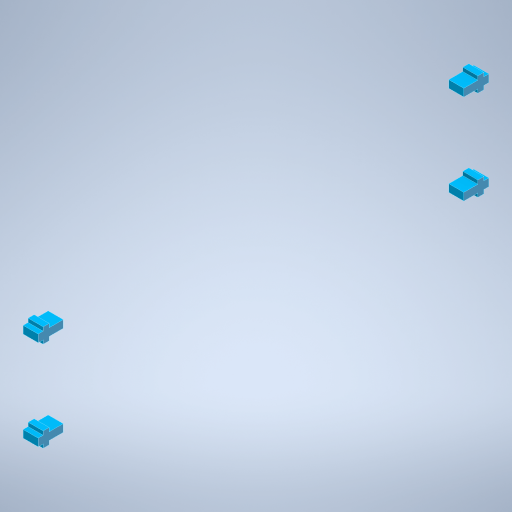
# Autodesk Inventor part: передняя стенка
Saved by Autodesk Inventor 2024.2 (Build 282272000, 272)
## iProperties
Created: 2025-11-20
Part Number: передняя стенка
Material: Типовые
Document SubType Name: Modeling
Designer: Zakhar
Density: 1 g/cm^3
Appearance: Небесно-голубой — нейтральный
Mass: 95.616 g
Surface Area: 351.84 cm^2
Volume: 95.616 cm^3
Author: Zakhar
Autodesk Inventor part; units mm, degrees
ref_plane "YZ Plane" through (0, 0, 0) normal (1, 0, 0) x (0, 1, 0)
ref_plane "XZ Plane" through (0, 0, 0) normal (0, 1, 0) x (-1, 0, 0)
ref_plane "XY Plane" through (0, 0, 0) normal (0, 0, 1) x (1, 0, 0)
sketch "Эскиз1" plane through (0, 0, 0) normal (1, 0, 0) x (0, 1, 0)
  line L0 (84, 90) -> (0, 90)
  line L1 (0, 90) -> (0, -90)
  line L2 (0, -90) -> (84, -90)
  line L3 (84, -90) -> (84, 90)
  line L4 (76, 90) -> (8, 90)
  line L5 (8, 90) -> (8, 96)
  line L6 (8, 96) -> (76, 96)
  line L7 (76, 96) -> (76, 90)
  line L8 (76, -90) -> (8, -90)
  line L9 (8, -90) -> (8, -96)
  line L10 (8, -96) -> (76, -96)
  line L11 (76, -96) -> (76, -90)
  line L12 (16, -96) -> (16, -90)
  line L13 (32, -96) -> (32, -90)
  line L14 (68, -96) -> (68, -90)
  line L15 (52, -96) -> (52, -90)
  line L16 (16, 90) -> (16, 96)
  line L17 (32, 90) -> (32, 96)
  line L18 (68, 90) -> (68, 96)
  line L19 (52, 90) -> (52, 96)
  circle A0 centre (20, -59.5) radius 1.5
  circle A1 centre (20, -73.5) radius 1.5
  circle A2 centre (7, -59.5) radius 1.5
  circle A3 centre (7, -73.5) radius 1.5
  line L20 (20, -59.5) -> (0, -59.5) construction
  line L21 (7, -59.5) -> (7, -73.5) construction
  line L22 (20, -73.5) -> (0, -73.5) construction
  point P0 (0, 0)
  point P1 (76, 93)
  point P2 (8, 93)
  point P3 (8, -90)
  point P4 (68, -93)
  point P5 (76, -93)
  point P6 (52, -93)
  point P7 (16, -93)
  point P8 (8, -93)
  point P9 (32, -93)
  point P10 (68, 93)
  point P11 (52, 93)
  point P12 (16, 93)
  point P13 (32, 93)
  dimension "d0" = 180
  dimension "d1" = 84
  dimension "d2" = 90
  dimension "d3" = 0
  dimension "d4" = 6
  dimension "d5" = 8
  dimension "d6" = 8
  dimension "d7" = 6
  dimension "d40" = 8
  dimension "d41" = 16
  dimension "d42" = 8
  dimension "d43" = 16
  dimension "d44" = 8
  dimension "d45" = 16
  dimension "d46" = 16
  dimension "d47" = 8
  dimension "d76" = 14
  dimension "d77" = 3
  dimension "d78" = 3
  dimension "d79" = 20
  dimension "d80" = 20
  dimension "d81" = 3
  dimension "d82" = 3
  dimension "d83" = 13
  dimension "d84" = 13
  dimension "d85" = 16.5
  constraints: 46 end point, 24 point on line, 13 perpendicular, 12 midpoint, 6 parallel, 4 centre point, 3 horizontal
  measures "d0" distance of L0.end L1.end
  measures "d1" distance of L0.start L0.end
  measures "d2" distance from line of point (0, 0) L2
  measures "d3" distance from line of L1 point (0, 0)
  measures "d4" distance of L6.end L4.start
  measures "d5" horizontal distance of L0.start point (76, 93)
  measures "d6" horizontal distance of L0.end point (8, 93)
  measures "d7" distance between parallel lines of L2 L10
  measures "d40" distance of point (68, -93) point (76, -93)
  measures "d41" distance of point (52, -93) point (68, -93)
  measures "d42" distance of point (16, -93) point (8, -93)
  measures "d43" distance of point (32, -93) point (16, -93)
  measures "d44" distance of point (76, 93) point (68, 93)
  measures "d45" distance of point (52, 93) point (68, 93)
  measures "d46" distance of point (16, 93) point (32, 93)
  measures "d47" distance of point (8, 93) point (16, 93)
  measures "d76" distance of L22.start L20.start
  measures "d77" diameter of A0
  measures "d78" diameter of A1
  measures "d79" distance from line of L1 L20.start
  measures "d80" distance from line of L1 L22.start
  measures "d81" diameter of A3
  measures "d82" diameter of A2
  measures "d83" distance of L20.start L21.start
  measures "d84" distance of L22.start L21.end
  measures "d85" distance from line of L8 L22.start
extrude "Выдавливание1" add sketch "Эскиз1" along normal blind 6 contours L3 L2 L1 L0 | L0 L18 L6 L7 | L11 L10 L14 L2 | L0 L17 L6 L19 | L15 L10 L13 L2 | L0 L5 L6 L16 | L12 L10 L9 L2
sketch "Эскиз4" plane through (0, 84, 90) normal (0, 1, 0) x (1, 0, 0)
  circle A0 centre (3, 5) radius 1.5
  circle A1 centre (3, 175) radius 1.5
  line L0 (0, 0) -> (6, 0)
  line L1 (6, 180) -> (6, 0)
  line L2 (0, 180) -> (6, 180)
  line L3 (6, 180) -> (6, 0) projected
  line L4 (0, 0) -> (6, 0) projected
  line L5 (0, 180) -> (6, 180) projected
  point P0 (0, 90)
  point P1 (3, 0)
  dimension "d30" = 3
  dimension "d31" = 3
  dimension "d32" = 5
  dimension "d33" = 3
  dimension "d34" = 5
  dimension "d35" = 3
  dimension "d36" = 6
  dimension "d37" = 6
  constraints: 6 end point, 3 collinear, 2 centre point, 1 midpoint
  measures "d30" diameter of A1
  measures "d31" diameter of A0
  measures "d32" distance of point (3, 0) A0.centre
  measures "d33" distance from line of L1 A0.centre
  measures "d34" distance from line of L2 A1.centre
  measures "d35" distance from line of L1 A1.centre
  measures "d36" distance of L2.start L1.start
  measures "d37" distance of L0.start L0.end
extrude "Выдавливание4" cut sketch "Эскиз4" against normal blind 4
sketch "Эскиз6" plane through (6, 0, 0) normal (1, 0, 0) x (0, 0, -1)
  line L0 (-90, 8) -> (-90, 0) projected
  line L1 (-90, 0) -> (-70, 0)
  line L2 (-70, 0) -> (-70, -6)
  line L3 (-70, -6) -> (-90, -6)
  line L4 (-90, -6) -> (-90, 0)
  line L5 (-90, 0) -> (90, 0) projected
  line L6 (-50, 0) -> (-30, 0)
  line L7 (-30, 0) -> (-30, -6)
  line L8 (-30, -6) -> (-50, -6)
  line L9 (-50, -6) -> (-50, 0)
  line L10 (30, 0) -> (50, 0)
  line L11 (50, 0) -> (50, -6)
  line L12 (50, -6) -> (30, -6)
  line L13 (30, -6) -> (30, 0)
  line L14 (90, 0) -> (70, 0)
  line L15 (70, 0) -> (70, -6)
  line L16 (70, -6) -> (90, -6)
  line L17 (90, -6) -> (90, 0)
  point P0 (0, 0)
  point P1 (-80, -6)
  point P2 (-50, -3)
  point P3 (-70, -3)
  point P4 (-30, -3)
  point P5 (90, -3)
  point P6 (70, -3)
  point P7 (50, -3)
  dimension "d48" = 6
  dimension "d49" = 6
  dimension "d50" = 6
  dimension "d51" = 20
  dimension "d52" = 20
  dimension "d53" = 20
  dimension "d54" = 20
  dimension "d55" = 20
  dimension "d56" = 20
  constraints: 32 end point, 8 parallel, 7 midpoint, 4 horizontal, 4 perpendicular, 3 point on line
  measures "d48" distance from line of L5 point (-80, -6)
  measures "d49" distance of L6.end L7.end
  measures "d50" distance of L12.end L10.start
  measures "d51" distance of L2.end L3.end
  measures "d52" distance of point (-50, -3) point (-70, -3)
  measures "d53" distance of point (-30, -3) point (-50, -3)
  measures "d54" distance of point (90, -3) point (70, -3)
  measures "d55" distance of point (70, -3) point (50, -3)
  measures "d56" distance from line of point (50, -3) L13
extrude "Выдавливание5" add sketch "Эскиз6" against normal blind 6
sketch "Эскиз8" plane through (0, 0, 0) normal (-1, 0, 0) x (0, 0, 1)
  line L0 (-26, 74) -> (-3, 74)
  line L1 (-3, 74) -> (-3, 62)
  line L2 (-3, 62) -> (-26, 62)
  line L3 (-26, 62) -> (-26, 74)
  circle A0 centre (-28.25, 71.5) radius 1.25
  circle A1 centre (-28.25, 64.5) radius 1.25
  circle A2 centre (-0.75, 71.5) radius 1.25
  circle A3 centre (-0.75, 64.5) radius 1.25
  line L4 (-90, 84) -> (90, 84) projected
  line L5 (-96, 68) -> (-96, 76) projected
  point P0 (0, 0)
  point P1 (-26, 68)
  dimension "d86" = 23
  dimension "d87" = 12
  dimension "d88" = 2.5
  dimension "d89" = 2.5
  dimension "d90" = 2.5
  dimension "d91" = 2.5
  dimension "d92" = 27.5
  dimension "d93" = 2.5
  dimension "d94" = 7
  dimension "d95" = 2.25
  dimension "d96" = 7
  dimension "d97" = 27.5
  dimension "d98" = 10
  dimension "d99" = 2.5
  dimension "d100" = 70
  dimension "d101" = 1
  constraints: 8 end point, 4 centre point, 2 parallel, 1 horizontal, 1 midpoint, 1 perpendicular
  measures "d86" distance of L1.end L2.end
  measures "d87" distance of L0.end L1.end
  measures "d88" diameter of A2
  measures "d89" diameter of A3
  measures "d90" diameter of A0
  measures "d91" diameter of A1
  measures "d92" distance of A2.centre A0.centre
  measures "d93" distance from line of L0 A0.centre
  measures "d94" distance of A1.centre A0.centre
  measures "d95" distance from line of A0.centre L3
  measures "d96" distance of A2.centre A3.centre
  measures "d97" distance of A1.centre A3.centre
  measures "d98" distance between parallel lines of L4 L0
  measures "d99" distance from line of L0 A2.centre
  measures "d100" distance from line of L5 point (-26, 68)
  measures "d101" distance edge to line of A3 L1
extrude "Выдавливание7" cut sketch "Эскиз8" against normal blind 10
sketch "Эскиз9" plane through (0, 0, 0) normal (-1, 0, 0) x (0, 0, 1)
  circle A0 centre (-39.4994, 58.5005) radius 1.5 projected
  circle A1 centre (10.5006, 58.4986) radius 1.5 projected
  circle A2 centre (-39.4994, 58.5005) radius 1.5
  circle A3 centre (10.5006, 58.4986) radius 1.5
  point P0 (0, 0)
  constraints: 2 centre point, 2 coincident, 2 concentric
extrude "Выдавливание8" cut sketch "Эскиз9" against normal blind 10
sketch "Эскиз10" plane through (0, 0, 0) normal (-1, 0, 0) x (0, 0, 1)
  line L0 (90, 61.5) -> (80, 61.5)
  line L1 (80, 61.5) -> (80, 58.5)
  line L2 (80, 58.5) -> (90, 58.5)
  line L3 (90, 58.5) -> (90, 61.5)
  line L4 (85.6, 57) -> (88, 57)
  line L5 (88, 57) -> (88, 63)
  line L6 (88, 63) -> (85.6, 63)
  line L7 (85.6, 63) -> (85.6, 57)
  line L8 (90, 25.5) -> (80, 25.5)
  line L9 (80, 25.5) -> (80, 22.5)
  line L10 (80, 22.5) -> (90, 22.5)
  line L11 (90, 22.5) -> (90, 25.5)
  line L12 (85.6, 27) -> (88, 27)
  line L13 (88, 27) -> (88, 21)
  line L14 (88, 21) -> (85.6, 21)
  line L15 (85.6, 21) -> (85.6, 27)
  circle A0 centre (10.5006, 58.4986) radius 1.5 projected
  circle A1 centre (-39.4994, 58.5005) radius 1.5 projected
  circle A2 centre (-28.25, 64.5) radius 1.25 projected
  circle A3 centre (-0.75, 71.5) radius 1.25 projected
  circle A4 centre (-28.25, 71.5) radius 1.25 projected
  circle A5 centre (-0.75, 64.5) radius 1.25 projected
  line L16 (-26, 74) -> (-26, 62) projected
  line L17 (-26, 62) -> (-3, 62) projected
  line L18 (-3, 62) -> (-3, 74) projected
  line L19 (-3, 74) -> (-26, 74) projected
  circle A6 centre (-73.5, 7) radius 1.5 projected
  circle A7 centre (-59.5, 7) radius 1.5 projected
  circle A8 centre (-73.5, 20) radius 1.5 projected
  circle A9 centre (-59.5, 20) radius 1.5 projected
  line L20 (90, 52) -> (96, 52) projected
  line L21 (96, 52) -> (96, 32) projected
  line L22 (96, 32) -> (90, 32) projected
  line L23 (90, 32) -> (90, 16) projected
  line L24 (90, 16) -> (96, 16) projected
  line L25 (96, 16) -> (96, 8) projected
  line L26 (96, 8) -> (90, 8) projected
  line L27 (90, 8) -> (90, -6) projected
  line L28 (90, -6) -> (70, -6) projected
  line L29 (70, -6) -> (70, 0) projected
  line L30 (70, 0) -> (50, 0) projected
  line L31 (50, 0) -> (50, -6) projected
  line L32 (50, -6) -> (30, -6) projected
  line L33 (30, -6) -> (30, 0) projected
  line L34 (30, 0) -> (-30, 0) projected
  line L35 (-30, 0) -> (-30, -6) projected
  line L36 (-30, -6) -> (-50, -6) projected
  line L37 (-50, -6) -> (-50, 0) projected
  line L38 (-50, 0) -> (-70, 0) projected
  line L39 (-70, 0) -> (-70, -6) projected
  line L40 (-70, -6) -> (-90, -6) projected
  line L41 (-90, -6) -> (-90, 8) projected
  line L42 (-90, 8) -> (-96, 8) projected
  line L43 (-96, 8) -> (-96, 16) projected
  line L44 (-96, 16) -> (-90, 16) projected
  line L45 (-90, 16) -> (-90, 32) projected
  line L46 (-90, 32) -> (-96, 32) projected
  line L47 (-96, 32) -> (-96, 52) projected
  line L48 (-96, 52) -> (-90, 52) projected
  line L49 (-90, 52) -> (-90, 68) projected
  line L50 (-90, 68) -> (-96, 68) projected
  line L51 (-96, 68) -> (-96, 76) projected
  line L52 (-96, 76) -> (-90, 76) projected
  line L53 (-90, 76) -> (-90, 84) projected
  line L54 (-90, 84) -> (90, 84) projected
  line L55 (90, 84) -> (90, 76) projected
  line L56 (90, 76) -> (96, 76) projected
  line L57 (96, 76) -> (96, 68) projected
  line L58 (96, 68) -> (90, 68) projected
  line L59 (90, 68) -> (90, 52) projected
  circle A10 centre (10.5006, 58.4986) radius 1.5 projected
  circle A11 centre (-39.4994, 58.5005) radius 1.5 projected
  circle A12 centre (-28.25, 64.5) radius 1.25 projected
  circle A13 centre (-0.75, 71.5) radius 1.25 projected
  circle A14 centre (-28.25, 71.5) radius 1.25 projected
  circle A15 centre (-0.75, 64.5) radius 1.25 projected
  line L60 (-26, 74) -> (-26, 62) projected
  line L61 (-26, 62) -> (-3, 62) projected
  line L62 (-3, 62) -> (-3, 74) projected
  line L63 (-3, 74) -> (-26, 74) projected
  circle A16 centre (-73.5, 7) radius 1.5 projected
  circle A17 centre (-59.5, 7) radius 1.5 projected
  circle A18 centre (-73.5, 20) radius 1.5 projected
  circle A19 centre (-59.5, 20) radius 1.5 projected
  line L64 (90, 52) -> (96, 52) projected
  line L65 (96, 52) -> (96, 32) projected
  line L66 (96, 32) -> (90, 32) projected
  line L67 (90, 32) -> (90, 16) projected
  line L68 (90, 16) -> (96, 16) projected
  line L69 (96, 16) -> (96, 8) projected
  line L70 (96, 8) -> (90, 8) projected
  line L71 (90, 8) -> (90, -6) projected
  line L72 (90, -6) -> (70, -6) projected
  line L73 (70, -6) -> (70, 0) projected
  line L74 (70, 0) -> (50, 0) projected
  line L75 (50, 0) -> (50, -6) projected
  line L76 (50, -6) -> (30, -6) projected
  line L77 (30, -6) -> (30, 0) projected
  line L78 (30, 0) -> (-30, 0) projected
  line L79 (-30, 0) -> (-30, -6) projected
  line L80 (-30, -6) -> (-50, -6) projected
  line L81 (-50, -6) -> (-50, 0) projected
  line L82 (-50, 0) -> (-70, 0) projected
  line L83 (-70, 0) -> (-70, -6) projected
  line L84 (-70, -6) -> (-90, -6) projected
  line L85 (-90, -6) -> (-90, 8) projected
  line L86 (-90, 8) -> (-96, 8) projected
  line L87 (-96, 8) -> (-96, 16) projected
  line L88 (-96, 16) -> (-90, 16) projected
  line L89 (-90, 16) -> (-90, 32) projected
  line L90 (-90, 32) -> (-96, 32) projected
  line L91 (-96, 32) -> (-96, 52) projected
  line L92 (-96, 52) -> (-90, 52) projected
  line L93 (-90, 52) -> (-90, 68) projected
  line L94 (-90, 68) -> (-96, 68) projected
  line L95 (-96, 68) -> (-96, 76) projected
  line L96 (-96, 76) -> (-90, 76) projected
  line L97 (-90, 76) -> (-90, 84) projected
  line L98 (-90, 84) -> (90, 84) projected
  line L99 (90, 84) -> (90, 76) projected
  line L100 (90, 76) -> (96, 76) projected
  line L101 (96, 76) -> (96, 68) projected
  line L102 (96, 68) -> (90, 68) projected
  line L103 (90, 68) -> (90, 52) projected
  circle A20 centre (10.5006, 58.4986) radius 1.5 projected
  circle A21 centre (-39.4994, 58.5005) radius 1.5 projected
  circle A22 centre (-28.25, 64.5) radius 1.25 projected
  circle A23 centre (-0.75, 71.5) radius 1.25 projected
  circle A24 centre (-28.25, 71.5) radius 1.25 projected
  circle A25 centre (-0.75, 64.5) radius 1.25 projected
  line L104 (-3, 74) -> (-3, 62) projected
  line L105 (-3, 62) -> (-26, 62) projected
  line L106 (-26, 62) -> (-26, 74) projected
  line L107 (-26, 74) -> (-3, 74) projected
  line L108 (96, 52) -> (96, 32) projected
  line L109 (90, 52) -> (96, 52) projected
  line L110 (90, 68) -> (90, 52) projected
  line L111 (96, 68) -> (90, 68) projected
  line L112 (96, 76) -> (96, 68) projected
  line L113 (90, 76) -> (96, 76) projected
  line L114 (90, 84) -> (90, 76) projected
  line L115 (-90, 84) -> (90, 84) projected
  line L116 (-90, 76) -> (-90, 84) projected
  line L117 (-96, 76) -> (-90, 76) projected
  line L118 (-96, 68) -> (-96, 76) projected
  line L119 (-90, 68) -> (-96, 68) projected
  line L120 (-90, 52) -> (-90, 68) projected
  line L121 (-96, 52) -> (-90, 52) projected
  line L122 (-96, 32) -> (-96, 52) projected
  line L123 (-90, 32) -> (-96, 32) projected
  line L124 (-90, 16) -> (-90, 32) projected
  line L125 (-96, 16) -> (-90, 16) projected
  line L126 (-96, 8) -> (-96, 16) projected
  line L127 (-90, 8) -> (-96, 8) projected
  line L128 (-90, 8) -> (-90, -6) projected
  line L129 (-90, -6) -> (-70, -6) projected
  line L130 (-70, -6) -> (-70, 0) projected
  line L131 (-50, 0) -> (-70, 0) projected
  line L132 (-50, 0) -> (-50, -6) projected
  line L133 (-50, -6) -> (-30, -6) projected
  line L134 (-30, -6) -> (-30, 0) projected
  line L135 (30, 0) -> (-30, 0) projected
  line L136 (30, 0) -> (30, -6) projected
  line L137 (30, -6) -> (50, -6) projected
  line L138 (50, -6) -> (50, 0) projected
  line L139 (70, 0) -> (50, 0) projected
  line L140 (70, 0) -> (70, -6) projected
  line L141 (70, -6) -> (90, -6) projected
  line L142 (90, 8) -> (90, -6) projected
  line L143 (96, 8) -> (90, 8) projected
  line L144 (96, 16) -> (96, 8) projected
  line L145 (90, 16) -> (96, 16) projected
  line L146 (90, 32) -> (90, 16) projected
  line L147 (96, 32) -> (90, 32) projected
  circle A26 centre (-59.5, 20) radius 1.5 projected
  circle A27 centre (-73.5, 20) radius 1.5 projected
  circle A28 centre (-59.5, 7) radius 1.5 projected
  circle A29 centre (-73.5, 7) radius 1.5 projected
  line L148 (90, 68) -> (90, 52) projected
  line L149 (0, 84) -> (0, 0) construction
  line L150 (-90, 61.5) -> (-80, 61.5)
  line L151 (-80, 61.5) -> (-80, 58.5)
  line L152 (-80, 58.5) -> (-90, 58.5)
  line L153 (-90, 58.5) -> (-90, 61.5)
  line L154 (-85.6, 57) -> (-88, 57)
  line L155 (-88, 57) -> (-88, 63)
  line L156 (-88, 63) -> (-85.6, 63)
  line L157 (-85.6, 63) -> (-85.6, 57)
  line L158 (-90, 25.5) -> (-80, 25.5)
  line L159 (-80, 25.5) -> (-80, 22.5)
  line L160 (-80, 22.5) -> (-90, 22.5)
  line L161 (-90, 22.5) -> (-90, 25.5)
  line L162 (-85.6, 27) -> (-88, 27)
  line L163 (-88, 27) -> (-88, 21)
  line L164 (-88, 21) -> (-85.6, 21)
  line L165 (-85.6, 21) -> (-85.6, 27)
  line L166 (-90, 52) -> (-96, 52)
  line L167 (-96, 52) -> (-96, 32)
  line L168 (-96, 32) -> (-90, 32)
  line L169 (-90, 32) -> (-90, 16)
  line L170 (-90, 16) -> (-96, 16)
  line L171 (-90, 52) -> (-96, 52)
  line L172 (-96, 52) -> (-96, 32)
  line L173 (-96, 32) -> (-90, 32)
  line L174 (-90, 32) -> (-90, 16)
  line L175 (-90, 16) -> (-96, 16)
  line L176 (-96, 52) -> (-96, 32)
  line L177 (-90, 52) -> (-96, 52)
  line L178 (-90, 16) -> (-96, 16)
  line L179 (-90, 32) -> (-90, 16)
  line L180 (-96, 32) -> (-90, 32)
  point P0 (93, 68)
  point P1 (93, 52)
  point P2 (93, 32)
  point P3 (-93, 52)
  point P4 (-93, 32)
  point P5 (85.6, 22.5)
  point P6 (88, 22.5)
  point P7 (88, 25.5)
  point P8 (85.6, 25.5)
  point P9 (85.6, 58.5)
  point P10 (88, 58.5)
  point P11 (88, 61.5)
  point P12 (85.6, 61.5)
  point P13 (-85.6, 25.5)
  point P14 (-88, 25.5)
  point P15 (-88, 22.5)
  point P16 (-85.6, 22.5)
  point P17 (-85.6, 61.5)
  point P18 (-88, 61.5)
  point P19 (-88, 58.5)
  point P20 (-85.6, 58.5)
  dimension "d106" = 6
  dimension "d107" = 2.4
  dimension "d108" = 10
  dimension "d109" = 3
  dimension "d110" = 1.5
  dimension "d111" = 5.6
  dimension "d112" = 10
  dimension "d113" = 3
  dimension "d114" = 1.5
  dimension "d115" = 6
  dimension "d116" = 5.6
  dimension "d117" = 2.4
  dimension "d118" = 6.5
  dimension "d120" = 6.5
  constraints: 96 end point, 30 symmetric about line, 8 parallel, 5 perpendicular, 4 horizontal, 4 midpoint, 2 point on line, 1 collinear
  measures "d106" distance between parallel lines of L14 L12
  measures "d107" distance between parallel lines of L15 L13
  measures "d108" distance of L9.end L10.end
  measures "d109" distance between parallel lines of L8 L10
  measures "d110" distance between parallel lines of L10 L14
  measures "d111" distance between parallel lines of L9 L15
  measures "d112" distance of L1.end L2.end
  measures "d113" distance of L2.end L0.start
  measures "d114" distance between parallel lines of L0 L6
  measures "d115" distance of L4.end L5.end
  measures "d116" distance between parallel lines of L1 L7
  measures "d117" distance of L4.start L4.end
  measures "d118" distance from line of point (93, 68) L0
  measures "d120" distance from line of L8 point (93, 32)
extrude "Выдавливание9" cut sketch "Эскиз10" against normal blind 10 contours L0 L5 L6 L7 L1 L2 L4 L59 L20 L21 L22 L23 L8 L13 L12 L15 L9 L10 L14 L24 L25 L26 L27 L28 L29 L30 L31 L32 L33 L34 L35 L36 L37 L38 L39 L40 L41 L42 L43 L44 L45 L160 L163 L164 L165 L159 L158 L162 L46 L47 L48 L49 L152 L155 L154 L157 L151 L150 L156 L50 L51 L52 L53 L54 L55 L56 L57 L58 | A0 | A1 | A2 | A3 | A4 | A5 | L19 L18 L17 L16 | A6 | A7 | A8 | A9
equation "\"d2\" = 0.5 * d0"
equation "\"d42\" = d40"
equation "\"d43\" = d41"
equation "\"d44\" = d40"
equation "\"d45\" = d41"
equation "\"d46\" = d41"
equation "\"d47\" = d40"
equation "\"d52\" = d51"
equation "\"d53\" = d51"
equation "\"d54\" = d51"
equation "\"d55\" = d51"
equation "\"d56\" = d51"
equation "\"d89\" = d88"
equation "\"d90\" = d88"
equation "\"d91\" = d88"
